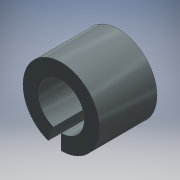
# Autodesk Inventor part: Clamp
Saved by Autodesk Inventor 2016 (Build 200138000, 138)
## iProperties
Created: 2016-04-20
Part Number: Clamp
Material: Generic
Document SubType Name: Modeling
Designer: Andres
Density: 1 g/cm^3
Appearance: Iron Gray
Author: Andres
Autodesk Inventor part; units mm, degrees
ref_plane "YZ Plane" through (0, 0, 0) normal (1, 0, 0) x (0, 1, 0)
ref_plane "XZ Plane" through (0, 0, 0) normal (0, 1, 0) x (-1, 0, 0)
ref_plane "XY Plane" through (0, 0, 0) normal (0, 0, 1) x (1, 0, 0)
sketch "Sketch1" plane through (0, 0, 0) normal (1, 0, 0) x (0, 1, 0)
  line L0 (0, 0) -> (7.5, 0)
  line L1 (7.5, 0) -> (7.5, -2)
  line L2 (7.5, -2) -> (0, -2)
  line L3 (0, -2) -> (0, 0)
  line L4 (7.5, 3) -> (0, 3)
  dimension "d0" = 2
  dimension "d1" = 7.5
  dimension "d2" = 7.5
  dimension "d3" = 3
  dimension "d4" = 0
  constraints: 10 end point, 2 horizontal, 2 parallel, 1 perpendicular
  measures "d0" distance of L0.end L1.end
  measures "d1" distance of L1.end L2.end
  measures "d2" distance of L4.start L4.end
  measures "d3" distance between parallel lines of L4 L0
  measures "d4" distance from line of L4.start L1
revolve "Revolution1" add sketch "Sketch1" angle 340 about axis through (0, 7.5, 3) along (0, -1, 0)
body "Solid1"
